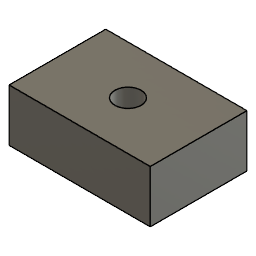
replay (Autodesk Fusion 360 design; units mm, degrees)
Autodesk Fusion 360 part; units mm, degrees
ref_plane "工作平面1" through (0, -8, 0) normal (0, 1, 0) x (0, 0, 1)
sketch "草图1" plane through (0, -8, 0) normal (0, 1, 0) x (1, 0, 0)
  line L0 (58, -42) -> (58, -5)
  line L1 (58, -5) -> (4, -5)
  line L2 (4, -5) -> (4, -42)
  line L3 (4, -42) -> (58, -42)
extrude "拉伸1" add sketch "草图1" along normal blind 20
sketch "草图2" plane through (0, 12, 0) normal (0, 1, 0) x (0, 0, 1)
  line L0 (42, 4) -> (42, 58)
  line L1 (42, 58) -> (5, 58)
  line L2 (5, 58) -> (5, 4)
  line L3 (5, 4) -> (42, 4)
  circle A0 centre (23.5, 31) radius 5
extrude "拉伸2" cut sketch "草图2" against normal through all contours A0
